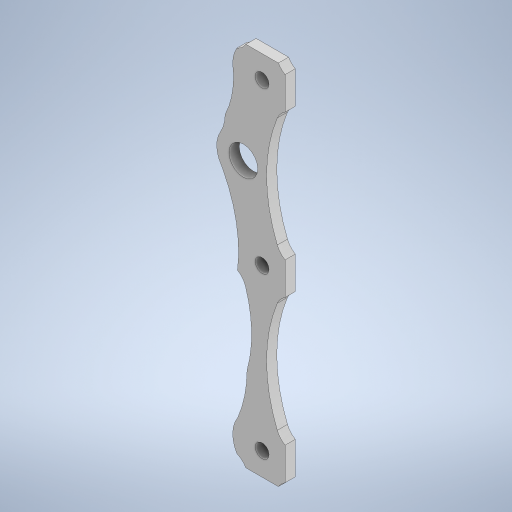
# Autodesk Inventor part: alta plate razz pi
Saved by Autodesk Inventor 2024 (Build 280153000, 153)
## iProperties
Created: 2024-04-18
Part Number: alta plate razz pi
Material: Generic
Document SubType Name: Modeling
Designer: Eli
Density: 1 g/cm^3
Appearance: Default
Author: Eli
Autodesk Inventor part; units mm, degrees
(part 1 of 2)
ref_plane "YZ Plane" through (0, 0, 0) normal (1, 0, 0) x (0, 1, 0)
ref_plane "XZ Plane" through (0, 0, 0) normal (0, 1, 0) x (-1, 0, 0)
ref_plane "XY Plane" through (0, 0, 0) normal (0, 0, 1) x (1, 0, 0)
sketch "Sketch1" plane through (0, 0, 0) normal (0, 0, 1) x (1, 0, 0)
  line L0 (57.15, -57.15) -> (-57.15, -57.15)
  line L1 (-57.15, -57.15) -> (-57.15, 57.15)
  line L2 (-57.15, 57.15) -> (57.15, 57.15)
  line L3 (57.15, 57.15) -> (57.15, -57.15)
  line L4 (0, 0) -> (-11.5551, 0)
  line L5 (0, 0) -> (0, -14.8829)
  arc A0 (-64.0069, -206.3369) -> (-62.0657, -206.8) centre (-62.0657, -202.5) ccw construction
  line L6 (-62.0657, -206.8) -> (-53.1, -206.8) construction
  arc A1 (-53.1, -206.8) -> (-51.8, -205.5) centre (-53.1, -205.5) ccw construction
  line L7 (-51.8, -205.5) -> (-51.8, -203.0447) construction
  arc A2 (-51.8, -203.0447) -> (-52.2776, -202.038) centre (-53.1, -203.0447) ccw construction
  arc A3 (-47.7224, -202.038) -> (-52.2776, -202.038) centre (-50, -199.25) ccw construction
  arc A4 (-47.7224, -202.038) -> (-48.2, -203.0447) centre (-46.9, -203.0447) ccw construction
  line L8 (-48.2, -203.0447) -> (-48.2, -205.5) construction
  arc A5 (-48.2, -205.5) -> (-46.9, -206.8) centre (-46.9, -205.5) ccw construction
  line L9 (-46.9, -206.8) -> (-43.2644, -206.8) construction
  arc A6 (-43.2644, -206.8) -> (-41.1799, -205.472) centre (-43.2644, -204.5) ccw construction
  line L10 (-41.1799, -205.472) -> (-36.3018, -195.0108) construction
  arc A7 (-34.6451, -192.9281) -> (-36.3018, -195.0108) centre (-31.1358, -197.4197) ccw construction
  line L11 (-34.6451, -192.9281) -> (-31.6765, -190.6087) construction
  arc A8 (-29.7064, -189.9304) -> (-31.6765, -190.6087) centre (-29.7064, -193.1304) ccw construction
  line L12 (-29.7064, -189.9304) -> (29.7064, -189.9304) construction
  arc A9 (31.6765, -190.6087) -> (29.7064, -189.9304) centre (29.7064, -193.1304) ccw construction
  line L13 (31.6765, -190.6087) -> (34.6451, -192.9281) construction
  arc A10 (36.3018, -195.0108) -> (34.6451, -192.9281) centre (31.1358, -197.4197) ccw construction
  line L14 (36.3018, -195.0108) -> (41.1799, -205.472) construction
  arc A11 (41.1799, -205.472) -> (43.2644, -206.8) centre (43.2644, -204.5) ccw construction
  line L15 (43.2644, -206.8) -> (46.9, -206.8) construction
  arc A12 (46.9, -206.8) -> (48.2, -205.5) centre (46.9, -205.5) ccw construction
  line L16 (48.2, -205.5) -> (48.2, -203.0447) construction
  arc A13 (48.2, -203.0447) -> (47.7224, -202.038) centre (46.9, -203.0447) ccw construction
  arc A14 (52.2776, -202.038) -> (47.7224, -202.038) centre (50, -199.25) ccw construction
  arc A15 (52.2776, -202.038) -> (51.8, -203.0447) centre (53.1, -203.0447) ccw construction
  line L17 (51.8, -203.0447) -> (51.8, -205.5) construction
  arc A16 (51.8, -205.5) -> (53.1, -206.8) centre (53.1, -205.5) ccw construction
  line L18 (53.1, -206.8) -> (62.0657, -206.8) construction
  arc A17 (62.0657, -206.8) -> (64.0069, -206.3369) centre (62.0657, -202.5) ccw construction
  arc A18 (65, -206.1) -> (64.0069, -206.3369) centre (65, -208.3) ccw construction
  line L19 (65, -206.1) -> (85, -206.1) construction
  arc A19 (85.9931, -206.3369) -> (85, -206.1) centre (85, -208.3) ccw construction
  arc A20 (85.9931, -206.3369) -> (87.9343, -206.8) centre (87.9343, -202.5) ccw construction
  line L20 (87.9343, -206.8) -> (96.9, -206.8) construction
  arc A21 (96.9, -206.8) -> (98.2, -205.5) centre (96.9, -205.5) ccw construction
  line L21 (98.2, -205.5) -> (98.2, -203.0447) construction
  arc A22 (98.2, -203.0447) -> (97.7224, -202.038) centre (96.9, -203.0447) ccw construction
  arc A23 (102.2776, -202.038) -> (97.7224, -202.038) centre (100, -199.25) ccw construction
  arc A24 (102.2776, -202.038) -> (101.8, -203.0447) centre (103.1, -203.0447) ccw construction
  line L22 (101.8, -203.0447) -> (101.8, -205.5) construction
  arc A25 (101.8, -205.5) -> (103.1, -206.8) centre (103.1, -205.5) ccw construction
  line L23 (103.1, -206.8) -> (112.0657, -206.8) construction
  arc A26 (112.0657, -206.8) -> (114.0069, -206.3369) centre (112.0657, -202.5) ccw construction
  arc A27 (115, -206.1) -> (114.0069, -206.3369) centre (115, -208.3) ccw construction
  line L24 (115, -206.1) -> (135, -206.1) construction
  arc A28 (135.9931, -206.3369) -> (135, -206.1) centre (135, -208.3) ccw construction
  arc A29 (135.9931, -206.3369) -> (137.9343, -206.8) centre (137.9343, -202.5) ccw construction
  line L25 (137.9343, -206.8) -> (146.9, -206.8) construction
  arc A30 (146.9, -206.8) -> (148.2, -205.5) centre (146.9, -205.5) ccw construction
  line L26 (148.2, -205.5) -> (148.2, -203.0447) construction
  arc A31 (148.2, -203.0447) -> (147.7224, -202.038) centre (146.9, -203.0447) ccw construction
  arc A32 (152.2776, -202.038) -> (147.7224, -202.038) centre (150, -199.25) ccw construction
  arc A33 (152.2776, -202.038) -> (151.8, -203.0447) centre (153.1, -203.0447) ccw construction
  line L27 (151.8, -203.0447) -> (151.8, -204.596) construction
  arc A34 (151.8, -204.596) -> (153.7003, -205.7491) centre (153.1, -204.596) ccw construction
  arc A35 (153.7003, -205.7491) -> (156.4467, -203.5758) centre (149.4058, -197.5) ccw construction
  arc A36 (203.5758, -156.4467) -> (156.4467, -203.5758) centre (500.278, -500.278) ccw construction
  arc A37 (203.5758, -156.4467) -> (205.7491, -153.7003) centre (197.5, -149.4058) ccw construction
  arc A38 (205.7491, -153.7003) -> (204.596, -151.8) centre (204.596, -153.1) ccw construction
  line L28 (204.596, -151.8) -> (203.0447, -151.8) construction
  arc A39 (203.0447, -151.8) -> (202.038, -152.2776) centre (203.0447, -153.1) ccw construction
  arc A40 (202.038, -147.7224) -> (202.038, -152.2776) centre (199.25, -150) ccw construction
  arc A41 (202.038, -147.7224) -> (203.0447, -148.2) centre (203.0447, -146.9) ccw construction
  line L29 (203.0447, -148.2) -> (205.5, -148.2) construction
  arc A42 (205.5, -148.2) -> (206.8, -146.9) centre (205.5, -146.9) ccw construction
  line L30 (206.8, -146.9) -> (206.8, -131.4343) construction
  arc A43 (206.8, -131.4343) -> (206.3369, -129.4931) centre (202.5, -131.4343) ccw construction
  arc A44 (206.1, -128.5) -> (206.3369, -129.4931) centre (208.3, -128.5) ccw construction
  line L31 (206.1, -128.5) -> (206.1, -108.5) construction
  arc A45 (206.3369, -107.5069) -> (206.1, -108.5) centre (208.3, -108.5) ccw construction
  arc A46 (206.3369, -107.5069) -> (206.8, -105.5657) centre (202.5, -105.5657) ccw construction
  line L32 (206.8, -105.5657) -> (206.8, -103.1) construction
  arc A47 (206.8, -103.1) -> (205.5, -101.8) centre (205.5, -103.1) ccw construction
  line L33 (205.5, -101.8) -> (203.0447, -101.8) construction
  arc A48 (203.0447, -101.8) -> (202.038, -102.2776) centre (203.0447, -103.1) ccw construction
  arc A49 (202.038, -97.7224) -> (202.038, -102.2776) centre (199.25, -100) ccw construction
  arc A50 (202.038, -97.7224) -> (203.0447, -98.2) centre (203.0447, -96.9) ccw construction
  line L34 (203.0447, -98.2) -> (205.5, -98.2) construction
  arc A51 (205.5, -98.2) -> (206.8, -96.9) centre (205.5, -96.9) ccw construction
  line L35 (206.8, -96.9) -> (206.8, -87.9343) construction
  arc A52 (206.8, -87.9343) -> (206.3369, -85.9931) centre (202.5, -87.9343) ccw construction
  arc A53 (206.1, -85) -> (206.3369, -85.9931) centre (208.3, -85) ccw construction
  line L36 (206.1, -85) -> (206.1, -65) construction
  arc A54 (206.3369, -64.0069) -> (206.1, -65) centre (208.3, -65) ccw construction
  arc A55 (206.3369, -64.0069) -> (206.8, -62.0657) centre (202.5, -62.0657) ccw construction
  line L37 (206.8, -62.0657) -> (206.8, -53.1) construction
  arc A56 (206.8, -53.1) -> (205.5, -51.8) centre (205.5, -53.1) ccw construction
  line L38 (205.5, -51.8) -> (203.0447, -51.8) construction
  arc A57 (203.0447, -51.8) -> (202.038, -52.2776) centre (203.0447, -53.1) ccw construction
  arc A58 (202.038, -47.7224) -> (202.038, -52.2776) centre (199.25, -50) ccw construction
  arc A59 (202.038, -47.7224) -> (203.0447, -48.2) centre (203.0447, -46.9) ccw construction
  line L39 (203.0447, -48.2) -> (205.5, -48.2) construction
  arc A60 (205.5, -48.2) -> (206.8, -46.9) centre (205.5, -46.9) ccw construction
  line L40 (206.8, -46.9) -> (206.8, -37.9343) construction
  arc A61 (206.8, -37.9343) -> (206.3369, -35.9931) centre (202.5, -37.9343) ccw construction
  arc A62 (206.1, -35) -> (206.3369, -35.9931) centre (208.3, -35) ccw construction
  line L41 (206.1, -35) -> (206.1, -15) construction
  arc A63 (206.3369, -14.0069) -> (206.1, -15) centre (208.3, -15) ccw construction
  arc A64 (206.3369, -14.0069) -> (206.8, -12.0657) centre (202.5, -12.0657) ccw construction
  line L42 (206.8, -12.0657) -> (206.8, -3.1) construction
  arc A65 (206.8, -3.1) -> (205.5, -1.8) centre (205.5, -3.1) ccw construction
  line L43 (205.5, -1.8) -> (203.0447, -1.8) construction
  arc A66 (203.0447, -1.8) -> (202.038, -2.2776) centre (203.0447, -3.1) ccw construction
  arc A67 (202.038, 2.2776) -> (202.038, -2.2776) centre (199.25, 0) ccw construction
  arc A68 (202.038, 2.2776) -> (203.0447, 1.8) centre (203.0447, 3.1) ccw construction
  line L44 (203.0447, 1.8) -> (205.5, 1.8) construction
  arc A69 (205.5, 1.8) -> (206.8, 3.1) centre (205.5, 3.1) ccw construction
  line L45 (206.8, 3.1) -> (206.8, 12.0657) construction
  arc A70 (206.8, 12.0657) -> (206.3369, 14.0069) centre (202.5, 12.0657) ccw construction
  arc A71 (206.1, 15) -> (206.3369, 14.0069) centre (208.3, 15) ccw construction
  line L46 (206.1, 15) -> (206.1, 35) construction
  arc A72 (206.3369, 35.9931) -> (206.1, 35) centre (208.3, 35) ccw construction
  arc A73 (206.3369, 35.9931) -> (206.8, 37.9343) centre (202.5, 37.9343) ccw construction
  line L47 (206.8, 37.9343) -> (206.8, 46.9) construction
  arc A74 (206.8, 46.9) -> (205.5, 48.2) centre (205.5, 46.9) ccw construction
  line L48 (205.5, 48.2) -> (203.0447, 48.2) construction
  arc A75 (203.0447, 48.2) -> (202.038, 47.7224) centre (203.0447, 46.9) ccw construction
  arc A76 (202.038, 52.2776) -> (202.038, 47.7224) centre (199.25, 50) ccw construction
  arc A77 (202.038, 52.2776) -> (203.0447, 51.8) centre (203.0447, 53.1) ccw construction
  line L49 (203.0447, 51.8) -> (205.5, 51.8) construction
  arc A78 (205.5, 51.8) -> (206.8, 53.1) centre (205.5, 53.1) ccw construction
  line L50 (206.8, 53.1) -> (206.8, 62.0657) construction
  arc A79 (206.8, 62.0657) -> (206.3369, 64.0069) centre (202.5, 62.0657) ccw construction
  arc A80 (206.1, 65) -> (206.3369, 64.0069) centre (208.3, 65) ccw construction
  line L51 (206.1, 65) -> (206.1, 85) construction
  arc A81 (206.3369, 85.9931) -> (206.1, 85) centre (208.3, 85) ccw construction
  arc A82 (206.3369, 85.9931) -> (206.8, 87.9343) centre (202.5, 87.9343) ccw construction
  line L52 (206.8, 87.9343) -> (206.8, 96.9) construction
  arc A83 (206.8, 96.9) -> (205.5, 98.2) centre (205.5, 96.9) ccw construction
  line L53 (205.5, 98.2) -> (203.0447, 98.2) construction
  arc A84 (203.0447, 98.2) -> (202.038, 97.7224) centre (203.0447, 96.9) ccw construction
  arc A85 (202.038, 102.2776) -> (202.038, 97.7224) centre (199.25, 100) ccw construction
  arc A86 (202.038, 102.2776) -> (203.0447, 101.8) centre (203.0447, 103.1) ccw construction
  line L54 (203.0447, 101.8) -> (205.5, 101.8) construction
  arc A87 (205.5, 101.8) -> (206.8, 103.1) centre (205.5, 103.1) ccw construction
  line L55 (206.8, 103.1) -> (206.8, 105.5657) construction
  arc A88 (206.8, 105.5657) -> (206.3369, 107.5069) centre (202.5, 105.5657) ccw construction
  arc A89 (206.1, 108.5) -> (206.3369, 107.5069) centre (208.3, 108.5) ccw construction
  line L56 (206.1, 108.5) -> (206.1, 128.5) construction
  arc A90 (206.3369, 129.4931) -> (206.1, 128.5) centre (208.3, 128.5) ccw construction
  arc A91 (206.3369, 129.4931) -> (206.8, 131.4343) centre (202.5, 131.4343) ccw construction
  line L57 (206.8, 131.4343) -> (206.8, 146.9) construction
  arc A92 (206.8, 146.9) -> (205.5, 148.2) centre (205.5, 146.9) ccw construction
  line L58 (205.5, 148.2) -> (203.0447, 148.2) construction
  arc A93 (203.0447, 148.2) -> (202.038, 147.7224) centre (203.0447, 146.9) ccw construction
  arc A94 (202.038, 152.2776) -> (202.038, 147.7224) centre (199.25, 150) ccw construction
  arc A95 (202.038, 152.2776) -> (203.0447, 151.8) centre (203.0447, 153.1) ccw construction
  line L59 (203.0447, 151.8) -> (204.596, 151.8) construction
  arc A96 (204.596, 151.8) -> (205.7491, 153.7003) centre (204.596, 153.1) ccw construction
  arc A97 (205.7491, 153.7003) -> (203.5758, 156.4467) centre (197.5, 149.4058) ccw construction
  arc A98 (156.4467, 203.5758) -> (203.5758, 156.4467) centre (500.278, 500.278) ccw construction
  arc A99 (156.4467, 203.5758) -> (153.7003, 205.7491) centre (149.4058, 197.5) ccw construction
  arc A100 (153.7003, 205.7491) -> (151.8, 204.596) centre (153.1, 204.596) ccw construction
  line L60 (151.8, 204.596) -> (151.8, 203.0447) construction
  arc A101 (151.8, 203.0447) -> (152.2776, 202.038) centre (153.1, 203.0447) ccw construction
  arc A102 (147.7224, 202.038) -> (152.2776, 202.038) centre (150, 199.25) ccw construction
  arc A103 (147.7224, 202.038) -> (148.2, 203.0447) centre (146.9, 203.0447) ccw construction
  line L61 (148.2, 203.0447) -> (148.2, 205.5) construction
  arc A104 (148.2, 205.5) -> (146.9, 206.8) centre (146.9, 205.5) ccw construction
  line L62 (146.9, 206.8) -> (137.9343, 206.8) construction
  arc A105 (137.9343, 206.8) -> (135.9931, 206.3369) centre (137.9343, 202.5) ccw construction
  arc A106 (135, 206.1) -> (135.9931, 206.3369) centre (135, 208.3) ccw construction
  line L63 (135, 206.1) -> (115, 206.1) construction
  arc A107 (114.0069, 206.3369) -> (115, 206.1) centre (115, 208.3) ccw construction
  arc A108 (114.0069, 206.3369) -> (112.0657, 206.8) centre (112.0657, 202.5) ccw construction
  line L64 (112.0657, 206.8) -> (103.1, 206.8) construction
  arc A109 (103.1, 206.8) -> (101.8, 205.5) centre (103.1, 205.5) ccw construction
  line L65 (101.8, 205.5) -> (101.8, 203.0447) construction
  arc A110 (101.8, 203.0447) -> (102.2776, 202.038) centre (103.1, 203.0447) ccw construction
  arc A111 (97.7224, 202.038) -> (102.2776, 202.038) centre (100, 199.25) ccw construction
  arc A112 (97.7224, 202.038) -> (98.2, 203.0447) centre (96.9, 203.0447) ccw construction
  line L66 (98.2, 203.0447) -> (98.2, 205.5) construction
  arc A113 (98.2, 205.5) -> (96.9, 206.8) centre (96.9, 205.5) ccw construction
  line L67 (96.9, 206.8) -> (87.9343, 206.8) construction
  arc A114 (87.9343, 206.8) -> (85.9931, 206.3369) centre (87.9343, 202.5) ccw construction
  arc A115 (85, 206.1) -> (85.9931, 206.3369) centre (85, 208.3) ccw construction
  line L68 (85, 206.1) -> (65, 206.1) construction
  arc A116 (64.0069, 206.3369) -> (65, 206.1) centre (65, 208.3) ccw construction
  arc A117 (64.0069, 206.3369) -> (62.0657, 206.8) centre (62.0657, 202.5) ccw construction
  line L69 (62.0657, 206.8) -> (53.1, 206.8) construction
  arc A118 (53.1, 206.8) -> (51.8, 205.5) centre (53.1, 205.5) ccw construction
  line L70 (51.8, 205.5) -> (51.8, 203.0447) construction
  arc A119 (51.8, 203.0447) -> (52.2776, 202.038) centre (53.1, 203.0447) ccw construction
  arc A120 (47.7224, 202.038) -> (52.2776, 202.038) centre (50, 199.25) ccw construction
  arc A121 (47.7224, 202.038) -> (48.2, 203.0447) centre (46.9, 203.0447) ccw construction
  line L71 (48.2, 203.0447) -> (48.2, 205.5) construction
  arc A122 (48.2, 205.5) -> (46.9, 206.8) centre (46.9, 205.5) ccw construction
  line L72 (46.9, 206.8) -> (37.9343, 206.8) construction
  arc A123 (37.9343, 206.8) -> (35.9931, 206.3369) centre (37.9343, 202.5) ccw construction
  arc A124 (35, 206.1) -> (35.9931, 206.3369) centre (35, 208.3) ccw construction
  line L73 (35, 206.1) -> (15, 206.1) construction
  arc A125 (14.0069, 206.3369) -> (15, 206.1) centre (15, 208.3) ccw construction
  arc A126 (14.0069, 206.3369) -> (12.0657, 206.8) centre (12.0657, 202.5) ccw construction
  line L74 (12.0657, 206.8) -> (3.1, 206.8) construction
  arc A127 (3.1, 206.8) -> (1.8, 205.5) centre (3.1, 205.5) ccw construction
  line L75 (1.8, 205.5) -> (1.8, 203.0447) construction
  arc A128 (1.8, 203.0447) -> (2.2776, 202.038) centre (3.1, 203.0447) ccw construction
  arc A129 (-2.2776, 202.038) -> (2.2776, 202.038) centre (0, 199.25) ccw construction
  arc A130 (-2.2776, 202.038) -> (-1.8, 203.0447) centre (-3.1, 203.0447) ccw construction
  line L76 (-1.8, 203.0447) -> (-1.8, 205.5) construction
  arc A131 (-1.8, 205.5) -> (-3.1, 206.8) centre (-3.1, 205.5) ccw construction
  line L77 (-3.1, 206.8) -> (-12.0657, 206.8) construction
  arc A132 (-12.0657, 206.8) -> (-14.0069, 206.3369) centre (-12.0657, 202.5) ccw construction
  arc A133 (-15, 206.1) -> (-14.0069, 206.3369) centre (-15, 208.3) ccw construction
  line L78 (-15, 206.1) -> (-35, 206.1) construction
  arc A134 (-35.9931, 206.3369) -> (-35, 206.1) centre (-35, 208.3) ccw construction
  arc A135 (-35.9931, 206.3369) -> (-37.9343, 206.8) centre (-37.9343, 202.5) ccw construction
  line L79 (-37.9343, 206.8) -> (-46.9, 206.8) construction
  arc A136 (-46.9, 206.8) -> (-48.2, 205.5) centre (-46.9, 205.5) ccw construction
  line L80 (-48.2, 205.5) -> (-48.2, 203.0447) construction
  arc A137 (-48.2, 203.0447) -> (-47.7224, 202.038) centre (-46.9, 203.0447) ccw construction
  arc A138 (-52.2776, 202.038) -> (-47.7224, 202.038) centre (-50, 199.25) ccw construction
  arc A139 (-52.2776, 202.038) -> (-51.8, 203.0447) centre (-53.1, 203.0447) ccw construction
  line L81 (-51.8, 203.0447) -> (-51.8, 205.5) construction
  arc A140 (-51.8, 205.5) -> (-53.1, 206.8) centre (-53.1, 205.5) ccw construction
  line L82 (-53.1, 206.8) -> (-62.0657, 206.8) construction
  arc A141 (-62.0657, 206.8) -> (-64.0069, 206.3369) centre (-62.0657, 202.5) ccw construction
  arc A142 (-65, 206.1) -> (-64.0069, 206.3369) centre (-65, 208.3) ccw construction
  line L83 (-65, 206.1) -> (-85, 206.1) construction
  arc A143 (-85.9931, 206.3369) -> (-85, 206.1) centre (-85, 208.3) ccw construction
  arc A144 (-85.9931, 206.3369) -> (-87.9343, 206.8) centre (-87.9343, 202.5) ccw construction
  line L84 (-87.9343, 206.8) -> (-96.9, 206.8) construction
  arc A145 (-96.9, 206.8) -> (-98.2, 205.5) centre (-96.9, 205.5) ccw construction
  line L85 (-98.2, 205.5) -> (-98.2, 203.0447) construction
  arc A146 (-98.2, 203.0447) -> (-97.7224, 202.038) centre (-96.9, 203.0447) ccw construction
  arc A147 (-102.2776, 202.038) -> (-97.7224, 202.038) centre (-100, 199.25) ccw construction
  arc A148 (-102.2776, 202.038) -> (-101.8, 203.0447) centre (-103.1, 203.0447) ccw construction
  line L86 (-101.8, 203.0447) -> (-101.8, 205.0441) construction
  arc A149 (-101.8, 205.0441) -> (-102.2153, 205.3211) centre (-102.1, 205.0441) ccw construction
  arc A150 (-102.2153, 205.3211) -> (-105.2513, 197.6241) centre (-100, 200) ccw construction
  arc A151 (-104.3, 193.2135) -> (-105.2513, 197.6241) centre (-115, 193.2135) ccw construction
  line L87 (-104.3, 193.2135) -> (-104.3, 171.5831) construction
  arc A152 (-158.4104, 151.7225) -> (-104.3, 171.5831) centre (-135, 171.5831) ccw construction
  arc A153 (-158.4104, 151.7225) -> (-163.9771, 154.3) centre (-163.9771, 147) ccw construction
  line L88 (-163.9771, 154.3) -> (-192.6198, 154.3) construction
  arc A154 (-196.9456, 155.2134) -> (-192.6198, 154.3) centre (-192.6198, 165) ccw construction
  arc A155 (-196.9456, 155.2134) -> (-204.2581, 152.7219) centre (-199.25, 150) ccw construction
  arc A156 (-204.5492, 152.2911) -> (-204.2581, 152.7219) centre (-206.6304, 154.0113) ccw construction
  arc A157 (-204.5492, 152.2911) -> (-204.318, 151.8) centre (-204.318, 152.1) ccw construction
  line L89 (-204.318, 151.8) -> (-203.0447, 151.8) construction
  arc A158 (-203.0447, 151.8) -> (-202.038, 152.2776) centre (-203.0447, 153.1) ccw construction
  arc A159 (-202.038, 147.7224) -> (-202.038, 152.2776) centre (-199.25, 150) ccw construction
  arc A160 (-202.038, 147.7224) -> (-203.0447, 148.2) centre (-203.0447, 146.9) ccw construction
  line L90 (-203.0447, 148.2) -> (-205.5, 148.2) construction
  arc A161 (-205.5, 148.2) -> (-206.8, 146.9) centre (-205.5, 146.9) ccw construction
  line L91 (-206.8, 146.9) -> (-206.8, 131.4343) construction
  arc A162 (-206.8, 131.4343) -> (-206.3369, 129.4931) centre (-202.5, 131.4343) ccw construction
  arc A163 (-206.1, 128.5) -> (-206.3369, 129.4931) centre (-208.3, 128.5) ccw construction
  line L92 (-206.1, 128.5) -> (-206.1, 108.5) construction
  arc A164 (-206.3369, 107.5069) -> (-206.1, 108.5) centre (-208.3, 108.5) ccw construction
  arc A165 (-206.3369, 107.5069) -> (-206.8, 105.5657) centre (-202.5, 105.5657) ccw construction
  line L93 (-206.8, 105.5657) -> (-206.8, 103.1) construction
  arc A166 (-206.8, 103.1) -> (-205.5, 101.8) centre (-205.5, 103.1) ccw construction
  line L94 (-205.5, 101.8) -> (-203.0447, 101.8) construction
  arc A167 (-203.0447, 101.8) -> (-202.038, 102.2776) centre (-203.0447, 103.1) ccw construction
  arc A168 (-202.038, 97.7224) -> (-202.038, 102.2776) centre (-199.25, 100) ccw construction
  arc A169 (-202.038, 97.7224) -> (-203.0447, 98.2) centre (-203.0447, 96.9) ccw construction
  line L95 (-203.0447, 98.2) -> (-205.5, 98.2) construction
  arc A170 (-205.5, 98.2) -> (-206.8, 96.9) centre (-205.5, 96.9) ccw construction
  line L96 (-206.8, 96.9) -> (-206.8, 87.9343) construction
  arc A171 (-206.8, 87.9343) -> (-206.3369, 85.9931) centre (-202.5, 87.9343) ccw construction
  arc A172 (-206.1, 85) -> (-206.3369, 85.9931) centre (-208.3, 85) ccw construction
  line L97 (-206.1, 85) -> (-206.1, 65) construction
  arc A173 (-206.3369, 64.0069) -> (-206.1, 65) centre (-208.3, 65) ccw construction
  arc A174 (-206.3369, 64.0069) -> (-206.8, 62.0657) centre (-202.5, 62.0657) ccw construction
  line L98 (-206.8, 62.0657) -> (-206.8, 53.1) construction
  arc A175 (-206.8, 53.1) -> (-205.5, 51.8) centre (-205.5, 53.1) ccw construction
  line L99 (-205.5, 51.8) -> (-203.0447, 51.8) construction
  arc A176 (-203.0447, 51.8) -> (-202.038, 52.2776) centre (-203.0447, 53.1) ccw construction
  arc A177 (-202.038, 47.7224) -> (-202.038, 52.2776) centre (-199.25, 50) ccw construction
  arc A178 (-202.038, 47.7224) -> (-203.0447, 48.2) centre (-203.0447, 46.9) ccw construction
  line L100 (-203.0447, 48.2) -> (-205.5, 48.2) construction
  arc A179 (-205.5, 48.2) -> (-206.8, 46.9) centre (-205.5, 46.9) ccw construction
  line L101 (-206.8, 46.9) -> (-206.8, 37.9343) construction
  arc A180 (-206.8, 37.9343) -> (-206.3369, 35.9931) centre (-202.5, 37.9343) ccw construction
  arc A181 (-206.1, 35) -> (-206.3369, 35.9931) centre (-208.3, 35) ccw construction
  line L102 (-206.1, 35) -> (-206.1, 15) construction
  arc A182 (-206.3369, 14.0069) -> (-206.1, 15) centre (-208.3, 15) ccw construction
  arc A183 (-206.3369, 14.0069) -> (-206.8, 12.0657) centre (-202.5, 12.0657) ccw construction
  line L103 (-206.8, 12.0657) -> (-206.8, 3.1) construction
  arc A184 (-206.8, 3.1) -> (-205.5, 1.8) centre (-205.5, 3.1) ccw construction
  line L104 (-205.5, 1.8) -> (-203.0447, 1.8) construction
  arc A185 (-203.0447, 1.8) -> (-202.038, 2.2776) centre (-203.0447, 3.1) ccw construction
  arc A186 (-202.038, -2.2776) -> (-202.038, 2.2776) centre (-199.25, 0) ccw construction
  arc A187 (-202.038, -2.2776) -> (-203.0447, -1.8) centre (-203.0447, -3.1) ccw construction
  line L105 (-203.0447, -1.8) -> (-205.5, -1.8) construction
  arc A188 (-205.5, -1.8) -> (-206.8, -3.1) centre (-205.5, -3.1) ccw construction
  line L106 (-206.8, -3.1) -> (-206.8, -12.0657) construction
  arc A189 (-206.8, -12.0657) -> (-206.3369, -14.0069) centre (-202.5, -12.0657) ccw construction
  arc A190 (-206.1, -15) -> (-206.3369, -14.0069) centre (-208.3, -15) ccw construction
  line L107 (-206.1, -15) -> (-206.1, -35) construction
  arc A191 (-206.3369, -35.9931) -> (-206.1, -35) centre (-208.3, -35) ccw construction
  arc A192 (-206.3369, -35.9931) -> (-206.8, -37.9343) centre (-202.5, -37.9343) ccw construction
  line L108 (-206.8, -37.9343) -> (-206.8, -46.9) construction
  arc A193 (-206.8, -46.9) -> (-205.5, -48.2) centre (-205.5, -46.9) ccw construction
  line L109 (-205.5, -48.2) -> (-203.0447, -48.2) construction
  arc A194 (-203.0447, -48.2) -> (-202.038, -47.7224) centre (-203.0447, -46.9) ccw construction
  arc A195 (-202.038, -52.2776) -> (-202.038, -47.7224) centre (-199.25, -50) ccw construction
  arc A196 (-202.038, -52.2776) -> (-203.0447, -51.8) centre (-203.0447, -53.1) ccw construction
  line L110 (-203.0447, -51.8) -> (-205.5, -51.8) construction
  arc A197 (-205.5, -51.8) -> (-206.8, -53.1) centre (-205.5, -53.1) ccw construction
  line L111 (-206.8, -53.1) -> (-206.8, -62.0657) construction
  arc A198 (-206.8, -62.0657) -> (-206.3369, -64.0069) centre (-202.5, -62.0657) ccw construction
  arc A199 (-206.1, -65) -> (-206.3369, -64.0069) centre (-208.3, -65) ccw construction
  line L112 (-206.1, -65) -> (-206.1, -85) construction
  arc A200 (-206.3369, -85.9931) -> (-206.1, -85) centre (-208.3, -85) ccw construction
  arc A201 (-206.3369, -85.9931) -> (-206.8, -87.9343) centre (-202.5, -87.9343) ccw construction
  line L113 (-206.8, -87.9343) -> (-206.8, -96.9) construction
  arc A202 (-206.8, -96.9) -> (-205.5, -98.2) centre (-205.5, -96.9) ccw construction
  line L114 (-205.5, -98.2) -> (-203.0447, -98.2) construction
  arc A203 (-203.0447, -98.2) -> (-202.038, -97.7224) centre (-203.0447, -96.9) ccw construction
  arc A204 (-202.038, -102.2776) -> (-202.038, -97.7224) centre (-199.25, -100) ccw construction
  arc A205 (-202.038, -102.2776) -> (-203.0447, -101.8) centre (-203.0447, -103.1) ccw construction
  line L115 (-203.0447, -101.8) -> (-205.5, -101.8) construction
  arc A206 (-205.5, -101.8) -> (-206.8, -103.1) centre (-205.5, -103.1) ccw construction
  line L116 (-206.8, -103.1) -> (-206.8, -105.5657) construction
  arc A207 (-206.8, -105.5657) -> (-206.3369, -107.5069) centre (-202.5, -105.5657) ccw construction
  arc A208 (-206.1, -108.5) -> (-206.3369, -107.5069) centre (-208.3, -108.5) ccw construction
  line L117 (-206.1, -108.5) -> (-206.1, -128.5) construction
  arc A209 (-206.3369, -129.4931) -> (-206.1, -128.5) centre (-208.3, -128.5) ccw construction
  arc A210 (-206.3369, -129.4931) -> (-206.8, -131.4343) centre (-202.5, -131.4343) ccw construction
  line L118 (-206.8, -131.4343) -> (-206.8, -146.9) construction
  arc A211 (-206.8, -146.9) -> (-205.5, -148.2) centre (-205.5, -146.9) ccw construction
  line L119 (-205.5, -148.2) -> (-203.0447, -148.2) construction
  arc A212 (-203.0447, -148.2) -> (-202.038, -147.7224) centre (-203.0447, -146.9) ccw construction
  arc A213 (-202.038, -152.2776) -> (-202.038, -147.7224) centre (-199.25, -150) ccw construction
  arc A214 (-202.038, -152.2776) -> (-203.0447, -151.8) centre (-203.0447, -153.1) ccw construction
  line L120 (-203.0447, -151.8) -> (-204.596, -151.8) construction
  arc A215 (-204.596, -151.8) -> (-205.7491, -153.7003) centre (-204.596, -153.1) ccw construction
  arc A216 (-205.7491, -153.7003) -> (-203.5758, -156.4467) centre (-197.5, -149.4058) ccw construction
  arc A217 (-156.4467, -203.5758) -> (-203.5758, -156.4467) centre (-500.278, -500.278) ccw construction
  arc A218 (-156.4467, -203.5758) -> (-153.7003, -205.7491) centre (-149.4058, -197.5) ccw construction
  arc A219 (-153.7003, -205.7491) -> (-151.8, -204.596) centre (-153.1, -204.596) ccw construction
  line L121 (-151.8, -204.596) -> (-151.8, -203.0447) construction
  arc A220 (-151.8, -203.0447) -> (-152.2776, -202.038) centre (-153.1, -203.0447) ccw construction
  arc A221 (-147.7224, -202.038) -> (-152.2776, -202.038) centre (-150, -199.25) ccw construction
  arc A222 (-147.7224, -202.038) -> (-148.2, -203.0447) centre (-146.9, -203.0447) ccw construction
  line L122 (-148.2, -203.0447) -> (-148.2, -205.5) construction
  arc A223 (-148.2, -205.5) -> (-146.9, -206.8) centre (-146.9, -205.5) ccw construction
  line L123 (-146.9, -206.8) -> (-137.9343, -206.8) construction
  arc A224 (-137.9343, -206.8) -> (-135.9931, -206.3369) centre (-137.9343, -202.5) ccw construction
  arc A225 (-135, -206.1) -> (-135.9931, -206.3369) centre (-135, -208.3) ccw construction
  line L124 (-135, -206.1) -> (-115, -206.1) construction
  arc A226 (-114.0069, -206.3369) -> (-115, -206.1) centre (-115, -208.3) ccw construction
  arc A227 (-114.0069, -206.3369) -> (-112.0657, -206.8) centre (-112.0657, -202.5) ccw construction
  line L125 (-112.0657, -206.8) -> (-103.1, -206.8) construction
  arc A228 (-103.1, -206.8) -> (-101.8, -205.5) centre (-103.1, -205.5) ccw construction
  line L126 (-101.8, -205.5) -> (-101.8, -203.0447) construction
  arc A229 (-101.8, -203.0447) -> (-102.2776, -202.038) centre (-103.1, -203.0447) ccw construction
  arc A230 (-97.7224, -202.038) -> (-102.2776, -202.038) centre (-100, -199.25) ccw construction
  arc A231 (-97.7224, -202.038) -> (-98.2, -203.0447) centre (-96.9, -203.0447) ccw construction
  line L127 (-98.2, -203.0447) -> (-98.2, -205.5) construction
  arc A232 (-98.2, -205.5) -> (-96.9, -206.8) centre (-96.9, -205.5) ccw construction
  line L128 (-96.9, -206.8) -> (-87.9343, -206.8) construction
  arc A233 (-87.9343, -206.8) -> (-85.9931, -206.3369) centre (-87.9343, -202.5) ccw construction
  arc A234 (-85, -206.1) -> (-85.9931, -206.3369) centre (-85, -208.3) ccw construction
  line L129 (-85, -206.1) -> (-65, -206.1) construction
  arc A235 (-64.0069, -206.3369) -> (-65, -206.1) centre (-65, -208.3) ccw construction
  circle A236 centre (0, 0) radius 16.7 projected
  arc A237 (-95.284, 192.1375) -> (-97.9043, 183.0505) centre (-52.919, 175) ccw construction
  arc A238 (-92.1375, 195.284) -> (-95.284, 192.1375) centre (-90, 190) ccw construction
  arc A239 (-57.8625, 195.284) -> (-92.1375, 195.284) centre (-75, 152.919) ccw construction
  arc A240 (-54.716, 192.1375) -> (-57.8625, 195.284) centre (-60, 190) ccw construction
  arc A241 (-51.531, 171.3004) -> (-54.716, 192.1375) centre (-97.081, 175) ccw construction
  arc A242 (-65.1933, 164.8787) -> (-51.531, 171.3004) centre (-60.2024, 172.0047) ccw construction
  line L130 (-65.1933, 164.8787) -> (-74.9534, 171.7143) construction
  arc A243 (-74.9534, 171.7143) -> (-78.4527, 172.8179) centre (-78.4527, 166.7179) ccw construction
  line L131 (-78.4527, 172.8179) -> (-89.3404, 172.8179) construction
  arc A244 (-97.9043, 183.0505) -> (-89.3404, 172.8179) centre (-89.3404, 181.5179) ccw construction
  arc A245 (-4.3, 165.4748) -> (-4.2294, 164.796) centre (-1, 165.4748) ccw construction
  spline S0 degree 3 poles (-4.2294, 164.796) (-3.9561, 163.4959) (-3.7785, 162.6294) (-3.9511, 160.1263) (-4.265, 159.1168) (-4.7061, 157.8883) knots -0.834043 -0.834043 -0.834043 -0.834043 -0.391594 -0.391594 0 0 0 0 construction
  arc A246 (-7.8625, 154.716) -> (-4.7057, 157.8881) centre (-10, 160) ccw construction
  arc A247 (-42.1375, 154.716) -> (-7.8625, 154.716) centre (-25, 197.081) ccw construction
  arc A248 (-45.284, 157.8625) -> (-42.1375, 154.716) centre (-40, 160) ccw construction
  arc A249 (-45.284, 192.1375) -> (-45.284, 157.8625) centre (-2.919, 175) ccw construction
  arc A250 (-42.1375, 195.284) -> (-45.284, 192.1375) centre (-40, 190) ccw construction
  arc A251 (-7.8625, 195.284) -> (-42.1375, 195.284) centre (-25, 152.919) ccw construction
  arc A252 (-4.716, 192.1375) -> (-7.8625, 195.284) centre (-10, 190) ccw construction
  arc A253 (-4.0769, 190.4642) -> (-4.716, 192.1375) centre (-47.081, 175) ccw construction
  spline S1 degree 3 poles (-4.0769, 190.4642) (-3.5122, 188.8935) (-3.1473, 187.619) (-3.1407, 185.5585) (-3.2145, 184.8443) (-3.591, 183.1727) (-3.7609, 182.7618) (-4.0541, 181.9333) knots -1.061398 -1.061398 -1.061398 -1.061398 -0.514056 -0.514056 -0.263625 -0.263625 0 0 0 0 construction
  arc A254 (-4.0541, 181.9333) -> (-4.3, 180.5) centre (0, 180.5) ccw construction
  line L132 (-4.3, 180.5) -> (-4.3, 165.4748) construction
  arc A255 (4.7057, 157.8881) -> (7.8625, 154.716) centre (10, 160) ccw construction
  spline S2 degree 3 poles (4.7061, 157.8883) (4.2708, 159.1004) (3.9515, 160.1229) (3.7784, 162.6286) (3.956, 163.4957) (4.2294, 164.796) knots -0.75207 -0.75207 -0.75207 -0.75207 -0.398606 -0.398606 0 0 0 0 construction
  arc A256 (4.2294, 164.796) -> (4.3, 165.4748) centre (1, 165.4748) ccw construction
  line L133 (4.3, 165.4748) -> (4.3, 180.5) construction
  arc A257 (4.3, 180.5) -> (4.0541, 181.9333) centre (0, 180.5) ccw construction
  spline S3 degree 3 poles (4.0541, 181.9333) (3.7622, 182.7581) (3.593, 183.1671) (3.1778, 185.0036) (3.1418, 185.7321) (3.1456, 187.6069) (3.5031, 188.8681) (4.0769, 190.4642) knots -0.820905 -0.820905 -0.820905 -0.820905 -0.675906 -0.675906 -0.50883 -0.50883 0 0 0 0 construction
  arc A258 (4.716, 192.1375) -> (4.0769, 190.4642) centre (47.081, 175) ccw construction
  arc A259 (7.8625, 195.284) -> (4.716, 192.1375) centre (10, 190) ccw construction
  arc A260 (42.1375, 195.284) -> (7.8625, 195.284) centre (25, 152.919) ccw construction
  arc A261 (45.284, 192.1375) -> (42.1375, 195.284) centre (40, 190) ccw construction
  arc A262 (45.284, 157.8625) -> (45.284, 192.1375) centre (2.919, 175) ccw construction
  arc A263 (42.1375, 154.716) -> (45.284, 157.8625) centre (40, 160) ccw construction
  arc A264 (7.8625, 154.716) -> (42.1375, 154.716) centre (25, 197.081) ccw construction
  arc A265 (57.8625, 195.284) -> (54.716, 192.1375) centre (60, 190) ccw construction
  arc A266 (92.1375, 195.284) -> (57.8625, 195.284) centre (75, 152.919) ccw construction
  arc A267 (95.284, 192.1375) -> (92.1375, 195.284) centre (90, 190) ccw construction
  arc A268 (95.284, 157.8625) -> (95.284, 192.1375) centre (52.919, 175) ccw construction
  arc A269 (92.1375, 154.716) -> (95.284, 157.8625) centre (90, 160) ccw construction
  arc A270 (57.8625, 154.716) -> (92.1375, 154.716) centre (75, 197.081) ccw construction
  arc A271 (54.716, 157.8625) -> (57.8625, 154.716) centre (60, 160) ccw construction
  arc A272 (54.716, 192.1375) -> (54.716, 157.8625) centre (97.081, 175) ccw construction
  arc A273 (107.8625, 195.284) -> (104.716, 192.1375) centre (110, 190) ccw construction
  arc A274 (142.1375, 195.284) -> (107.8625, 195.284) centre (125, 152.919) ccw construction
  arc A275 (145.284, 192.1375) -> (142.1375, 195.284) centre (140, 190) ccw construction
  arc A276 (145.284, 157.8625) -> (145.284, 192.1375) centre (102.919, 175) ccw construction
  arc A277 (142.1375, 154.716) -> (145.284, 157.8625) centre (140, 160) ccw construction
  arc A278 (107.8625, 154.716) -> (142.1375, 154.716) centre (125, 197.081) ccw construction
  arc A279 (104.716, 157.8625) -> (107.8625, 154.716) centre (110, 160) ccw construction
  arc A280 (104.716, 192.1375) -> (104.716, 157.8625) centre (147.081, 175) ccw construction
  arc A281 (151.4988, 171.7212) -> (154.716, 157.8625) centre (197.081, 175) ccw construction
  arc A282 (166.4392, 178.3841) -> (151.4988, 171.7212) centre (160.1763, 172.3454) ccw construction
  arc A283 (166.4392, 178.3841) -> (178.3841, 166.4392) centre (500.278, 500.278) ccw construction
  arc A284 (171.7212, 151.4988) -> (178.3841, 166.4392) centre (172.3454, 160.1763) ccw construction
  arc A285 (157.8625, 154.716) -> (171.7212, 151.4988) centre (175, 197.081) ccw construction
  arc A286 (154.716, 157.8625) -> (157.8625, 154.716) centre (160, 160) ccw construction
  arc A287 (181.1757, 148.1998) -> (157.8625, 145.284) centre (175, 102.919) ccw construction
  arc A288 (188.7, 139.5796) -> (181.1757, 148.1998) centre (180, 139.5796) ccw construction
  line L134 (188.7, 139.5796) -> (188.7, 137.0711) construction
  arc A289 (188.7, 137.0711) -> (189.9594, 134.0305) centre (193, 137.0711) ccw construction
  line L135 (189.9594, 134.0305) -> (196.9023, 127.0876) construction
  arc A290 (198.5651, 122.7803) -> (196.9023, 127.0876) centre (192.8718, 123.0571) ccw construction
  arc A291 (195.284, 107.8625) -> (198.5651, 122.7803) centre (152.919, 125) ccw construction
  arc A292 (192.1375, 104.716) -> (195.284, 107.8625) centre (190, 110) ccw construction
  arc A293 (168.9997, 101.7766) -> (192.1375, 104.716) centre (175, 147.081) ccw construction
  arc A294 (163.9859, 111.6056) -> (168.9997, 101.7766) centre (169.8794, 108.4186) ccw construction
  arc A295 (163.9859, 111.6056) -> (158.7814, 119.3988) centre (159.3239, 114.1267) ccw construction
  arc A296 (151.398, 126.2464) -> (158.7814, 119.3988) centre (158.0955, 126.0637) ccw construction
  arc A297 (154.716, 142.1375) -> (151.398, 126.2464) centre (197.081, 125) ccw construction
  arc A298 (157.8625, 145.284) -> (154.716, 142.1375) centre (160, 140) ccw construction
  line L136 (172.8179, 78.4527) -> (172.8179, 89.3404) construction
  arc A299 (183.0505, 97.9043) -> (172.8179, 89.3404) centre (181.5179, 89.3404) ccw construction
  arc A300 (192.1375, 95.284) -> (183.0505, 97.9043) centre (175, 52.919) ccw construction
  arc A301 (195.284, 92.1375) -> (192.1375, 95.284) centre (190, 90) ccw construction
  arc A302 (195.284, 57.8625) -> (195.284, 92.1375) centre (152.919, 75) ccw construction
  arc A303 (192.1375, 54.716) -> (195.284, 57.8625) centre (190, 60) ccw construction
  arc A304 (171.3004, 51.531) -> (192.1375, 54.716) centre (175, 97.081) ccw construction
  arc A305 (164.8787, 65.1933) -> (171.3004, 51.531) centre (172.0047, 60.2024) ccw construction
  line L137 (164.8787, 65.1933) -> (171.7143, 74.9534) construction
  arc A306 (171.7143, 74.9534) -> (172.8179, 78.4527) centre (166.7179, 78.4527) ccw construction
  arc A307 (128.4924, 148.4854) -> (107.8625, 145.284) centre (125, 102.919) ccw construction
  arc A308 (133.4107, 144.758) -> (128.4924, 148.4854) centre (128.0568, 142.802) ccw construction
  arc A309 (133.4107, 144.758) -> (139.1817, 140.7513) centre (139.1403, 146.8512) ccw construction
  arc A310 (147.7814, 133.7096) -> (139.1817, 140.7513) centre (139.2409, 132.0515) ccw construction
  arc A311 (145.284, 107.8625) -> (147.7814, 133.7096) centre (102.919, 125) ccw construction
  arc A312 (142.1375, 104.716) -> (145.284, 107.8625) centre (140, 110) ccw construction
  arc A313 (107.8625, 104.716) -> (142.1375, 104.716) centre (125, 147.081) ccw construction
  arc A314 (104.716, 107.8625) -> (107.8625, 104.716) centre (110, 110) ccw construction
  arc A315 (104.716, 142.1375) -> (104.716, 107.8625) centre (147.081, 125) ccw construction
  arc A316 (107.8625, 145.284) -> (104.716, 142.1375) centre (110, 140) ccw construction
  arc A317 (139.6902, 96.1936) -> (142.6797, 95.7) centre (142.6797, 105) ccw construction
  line L138 (142.6797, 95.7) -> (156, 95.7) construction
  arc A318 (160.7, 91) -> (156, 95.7) centre (156, 91) ccw construction
  line L139 (160.7, 91) -> (160.7, 82.9939) construction
  arc A319 (158.7642, 76.8556) -> (160.7, 82.9939) centre (150, 82.9939) ccw construction
  line L140 (158.7642, 76.8556) -> (144.6688, 56.7301) construction
  arc A320 (142.1375, 54.716) -> (144.6688, 56.7301) centre (140, 60) ccw construction
  arc A321 (107.8625, 54.716) -> (142.1375, 54.716) centre (125, 97.081) ccw construction
  arc A322 (104.716, 57.8625) -> (107.8625, 54.716) centre (110, 60) ccw construction
  arc A323 (104.716, 92.1375) -> (104.716, 57.8625) centre (147.081, 75) ccw construction
  arc A324 (107.8625, 95.284) -> (104.716, 92.1375) centre (110, 90) ccw construction
  arc A325 (139.6902, 96.1936) -> (107.8625, 95.284) centre (125, 52.919) ccw construction
  arc A326 (57.8625, 145.284) -> (54.716, 142.1375) centre (60, 140) ccw construction
  arc A327 (92.1375, 145.284) -> (57.8625, 145.284) centre (75, 102.919) ccw construction
  arc A328 (95.284, 142.1375) -> (92.1375, 145.284) centre (90, 140) ccw construction
  arc A329 (95.284, 107.8625) -> (95.284, 142.1375) centre (52.919, 125) ccw construction
  arc A330 (92.1375, 104.716) -> (95.284, 107.8625) centre (90, 110) ccw construction
  arc A331 (57.8625, 104.716) -> (92.1375, 104.716) centre (75, 147.081) ccw construction
  arc A332 (54.716, 107.8625) -> (57.8625, 104.716) centre (60, 110) ccw construction
  arc A333 (54.716, 142.1375) -> (54.716, 107.8625) centre (97.081, 125) ccw construction
  arc A334 (57.8625, 95.284) -> (54.716, 92.1375) centre (60, 90) ccw construction
  arc A335 (92.1375, 95.284) -> (57.8625, 95.284) centre (75, 52.919) ccw construction
  arc A336 (95.284, 92.1375) -> (92.1375, 95.284) centre (90, 90) ccw construction
  arc A337 (95.284, 57.8625) -> (95.284, 92.1375) centre (52.919, 75) ccw construction
  arc A338 (92.1375, 54.716) -> (95.284, 57.8625) centre (90, 60) ccw construction
  arc A339 (57.8625, 54.716) -> (92.1375, 54.716) centre (75, 97.081) ccw construction
  arc A340 (54.716, 57.8625) -> (57.8625, 54.716) centre (60, 60) ccw projected
  arc A341 (54.716, 92.1375) -> (54.716, 57.8625) centre (97.081, 75) ccw construction
  arc A342 (7.8625, 95.284) -> (4.716, 92.1375) centre (10, 90) ccw construction
  arc A343 (42.1375, 95.284) -> (7.8625, 95.284) centre (25, 52.919) ccw construction
  arc A344 (45.284, 92.1375) -> (42.1375, 95.284) centre (40, 90) ccw construction
  arc A345 (45.284, 57.8625) -> (45.284, 92.1375) centre (2.919, 75) ccw construction
  arc A346 (42.1375, 54.716) -> (45.284, 57.8625) centre (40, 60) ccw projected
  arc A347 (7.8625, 54.716) -> (42.1375, 54.716) centre (25, 97.081) ccw projected
  arc A348 (4.716, 57.8625) -> (7.8625, 54.716) centre (10, 60) ccw projected
  arc A349 (4.716, 92.1375) -> (4.716, 57.8625) centre (47.081, 75) ccw construction
  arc A350 (7.8625, 145.284) -> (4.716, 142.1375) centre (10, 140) ccw construction
  arc A351 (42.1375, 145.284) -> (7.8625, 145.284) centre (25, 102.919) ccw construction
  arc A352 (45.284, 142.1375) -> (42.1375, 145.284) centre (40, 140) ccw construction
  arc A353 (45.284, 107.8625) -> (45.284, 142.1375) centre (2.919, 125) ccw construction
  arc A354 (42.1375, 104.716) -> (45.284, 107.8625) centre (40, 110) ccw construction
  arc A355 (7.8625, 104.716) -> (42.1375, 104.716) centre (25, 147.081) ccw construction
  arc A356 (4.716, 107.8625) -> (7.8625, 104.716) centre (10, 110) ccw construction
  arc A357 (4.716, 142.1375) -> (4.716, 107.8625) centre (47.081, 125) ccw construction
  arc A358 (-42.1375, 145.284) -> (-45.284, 142.1375) centre (-40, 140) ccw construction
  arc A359 (-7.8625, 145.284) -> (-42.1375, 145.284) centre (-25, 102.919) ccw construction
  arc A360 (-4.716, 142.1375) -> (-7.8625, 145.284) centre (-10, 140) ccw construction
  arc A361 (-4.716, 107.8625) -> (-4.716, 142.1375) centre (-47.081, 125) ccw construction
  arc A362 (-7.8625, 104.716) -> (-4.716, 107.8625) centre (-10, 110) ccw construction
  arc A363 (-42.1375, 104.716) -> (-7.8625, 104.716) centre (-25, 147.081) ccw construction
  arc A364 (-45.284, 107.8625) -> (-42.1375, 104.716) centre (-40, 110) ccw construction
  arc A365 (-45.284, 142.1375) -> (-45.284, 107.8625) centre (-2.919, 125) ccw construction
  arc A366 (-104.2647, 147.0916) -> (-98.2473, 157.6646) centre (-135, 171.5831) ccw construction
  arc A367 (-93.8519, 160.7) -> (-98.2473, 157.6646) centre (-93.8519, 156) ccw construction
  line L141 (-93.8519, 160.7) -> (-82.9939, 160.7) construction
  arc A368 (-76.8556, 158.7642) -> (-82.9939, 160.7) centre (-82.9939, 150) ccw construction
  line L142 (-76.8556, 158.7642) -> (-56.7301, 144.6688) construction
  arc A369 (-54.716, 142.1375) -> (-56.7301, 144.6688) centre (-60, 140) ccw construction
  arc A370 (-54.716, 107.8625) -> (-54.716, 142.1375) centre (-97.081, 125) ccw construction
  arc A371 (-57.8625, 104.716) -> (-54.716, 107.8625) centre (-60, 110) ccw construction
  arc A372 (-92.1375, 104.716) -> (-57.8625, 104.716) centre (-75, 147.081) ccw construction
  arc A373 (-95.284, 107.8625) -> (-92.1375, 104.716) centre (-90, 110) ccw construction
  arc A374 (-98.3342, 130.0942) -> (-95.284, 107.8625) centre (-52.919, 125) ccw construction
  arc A375 (-98.3342, 130.0942) -> (-98.6167, 133.6242) centre (-107.5762, 131.1309) ccw construction
  arc A376 (-98.6167, 133.6242) -> (-103.3198, 140.3374) centre (-110.4664, 130.3266) ccw construction
  arc A377 (-104.2647, 147.0916) -> (-103.3198, 140.3374) centre (-100.589, 144.1626) ccw construction
  arc A378 (-139.0124, 132.4885) -> (-148.5963, 123.5598) centre (-139.9006, 123.8339) ccw construction
  arc A379 (-139.0124, 132.4885) -> (-114.9131, 137.8043) centre (-135, 171.5831) ccw construction
  arc A380 (-101.857, 131.579) -> (-114.9131, 137.8043) centre (-110.4664, 130.3266) ccw construction
  arc A381 (-104.716, 107.8625) -> (-101.857, 131.579) centre (-147.081, 125) ccw construction
  arc A382 (-107.8625, 104.716) -> (-104.716, 107.8625) centre (-110, 110) ccw construction
  arc A383 (-142.1375, 104.716) -> (-107.8625, 104.716) centre (-125, 147.081) ccw construction
  arc A384 (-145.284, 107.8625) -> (-142.1375, 104.716) centre (-140, 110) ccw construction
  arc A385 (-148.5963, 123.5598) -> (-145.284, 107.8625) centre (-102.919, 125) ccw construction
  arc A386 (-189.9594, 134.0305) -> (-188.7, 137.0711) centre (-193, 137.0711) ccw construction
  line L143 (-188.7, 137.0711) -> (-188.7, 139.5796) construction
  arc A387 (-181.1757, 148.1998) -> (-188.7, 139.5796) centre (-180, 139.5796) ccw construction
  arc A388 (-163.3591, 147.1115) -> (-181.1757, 148.1998) centre (-175, 102.919) ccw construction
  arc A389 (-152.8885, 136.6409) -> (-163.3591, 147.1115) centre (-167.1036, 132.8964) ccw construction
  arc A390 (-151.6379, 129.8385) -> (-152.8885, 136.6409) centre (-197.081, 125) ccw construction
  arc A391 (-160.289, 120.2174) -> (-151.6379, 129.8385) centre (-160.289, 128.9174) ccw construction
  line L144 (-160.289, 120.2174) -> (-167.8239, 120.2174) construction
  arc A392 (-167.8239, 120.2174) -> (-172.1372, 118.4308) centre (-167.8239, 114.1174) ccw construction
  line L145 (-172.1372, 118.4308) -> (-184.5985, 105.9695) construction
  arc A393 (-188.629, 104.3) -> (-184.5985, 105.9695) centre (-188.629, 110) ccw construction
  line L146 (-188.629, 104.3) -> (-190, 104.3) construction
  arc A394 (-195.284, 107.8625) -> (-190, 104.3) centre (-190, 110) ccw construction
  arc A395 (-198.5651, 122.7803) -> (-195.284, 107.8625) centre (-152.919, 125) ccw construction
  arc A396 (-196.9023, 127.0876) -> (-198.5651, 122.7803) centre (-192.8718, 123.0571) ccw construction
  line L147 (-196.9023, 127.0876) -> (-189.9594, 134.0305) construction
  arc A397 (-42.1375, 95.284) -> (-45.284, 92.1375) centre (-40, 90) ccw construction
  arc A398 (-7.8625, 95.284) -> (-42.1375, 95.284) centre (-25, 52.919) ccw construction
  arc A399 (-4.716, 92.1375) -> (-7.8625, 95.284) centre (-10, 90) ccw construction
  arc A400 (-4.716, 57.8625) -> (-4.716, 92.1375) centre (-47.081, 75) ccw construction
  arc A401 (-7.8625, 54.716) -> (-4.716, 57.8625) centre (-10, 60) ccw projected
  arc A402 (-42.1375, 54.716) -> (-7.8625, 54.716) centre (-25, 97.081) ccw projected
  arc A403 (-45.284, 57.8625) -> (-42.1375, 54.716) centre (-40, 60) ccw projected
  arc A404 (-45.284, 92.1375) -> (-45.284, 57.8625) centre (-2.919, 75) ccw construction
  arc A405 (-92.1375, 95.284) -> (-95.284, 92.1375) centre (-90, 90) ccw construction
  arc A406 (-57.8625, 95.284) -> (-92.1375, 95.284) centre (-75, 52.919) ccw construction
  arc A407 (-54.716, 92.1375) -> (-57.8625, 95.284) centre (-60, 90) ccw construction
  arc A408 (-54.716, 57.8625) -> (-54.716, 92.1375) centre (-97.081, 75) ccw construction
  arc A409 (-57.8625, 54.716) -> (-54.716, 57.8625) centre (-60, 60) ccw projected
  arc A410 (-92.1375, 54.716) -> (-57.8625, 54.716) centre (-75, 97.081) ccw construction
  arc A411 (-95.284, 57.8625) -> (-92.1375, 54.716) centre (-90, 60) ccw construction
  arc A412 (-95.284, 92.1375) -> (-95.284, 57.8625) centre (-52.919, 75) ccw construction
  arc A413 (-142.1375, 95.284) -> (-145.284, 92.1375) centre (-140, 90) ccw construction
  arc A414 (-107.8625, 95.284) -> (-142.1375, 95.284) centre (-125, 52.919) ccw construction
  arc A415 (-104.716, 92.1375) -> (-107.8625, 95.284) centre (-110, 90) ccw construction
  arc A416 (-104.716, 57.8625) -> (-104.716, 92.1375) centre (-147.081, 75) ccw construction
  arc A417 (-107.8625, 54.716) -> (-104.716, 57.8625) centre (-110, 60) ccw construction
  arc A418 (-142.1375, 54.716) -> (-107.8625, 54.716) centre (-125, 97.081) ccw construction
  arc A419 (-145.284, 57.8625) -> (-142.1375, 54.716) centre (-140, 60) ccw construction
  arc A420 (-145.284, 92.1375) -> (-145.284, 57.8625) centre (-102.919, 75) ccw construction
  arc A421 (-142.1375, 45.284) -> (-145.284, 42.1375) centre (-140, 40) ccw construction
  arc A422 (-107.8625, 45.284) -> (-142.1375, 45.284) centre (-125, 2.919) ccw construction
  arc A423 (-104.716, 42.1375) -> (-107.8625, 45.284) centre (-110, 40) ccw construction
  arc A424 (-104.716, 7.8625) -> (-104.716, 42.1375) centre (-147.081, 25) ccw construction
  arc A425 (-107.8625, 4.716) -> (-104.716, 7.8625) centre (-110, 10) ccw construction
  arc A426 (-142.1375, 4.716) -> (-107.8625, 4.716) centre (-125, 47.081) ccw construction
  arc A427 (-145.284, 7.8625) -> (-142.1375, 4.716) centre (-140, 10) ccw construction
  arc A428 (-145.284, 42.1375) -> (-145.284, 7.8625) centre (-102.919, 25) ccw construction
  arc A429 (-157.3723, 102.2164) -> (-161.9122, 105.7) centre (-161.9122, 101) ccw construction
  line L148 (-157.3723, 102.2164) -> (-154.5817, 91.8019) construction
  arc A430 (-154.716, 57.8625) -> (-154.5817, 91.8019) centre (-197.081, 75) ccw construction
  arc A431 (-157.8625, 54.716) -> (-154.716, 57.8625) centre (-160, 60) ccw construction
  arc A432 (-192.1375, 54.716) -> (-157.8625, 54.716) centre (-175, 97.081) ccw construction